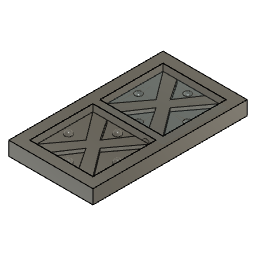
Verkefni_5_1 v3 (Autodesk Fusion 360 design; units mm, degrees)
Autodesk Fusion 360 part; units mm, degrees
sketch "Sketch1" plane through (0, 0, 0) normal (0, 0, 1) x (1, 0, 0)
  line L0 (-40, -40) -> (-10, 0)
  line L1 (-20, -40) -> (0, -10)
  line L2 (0, -10) -> (20, -40)
  line L3 (-40, -40) -> (-20, -40)
  line L4 (10, 0) -> (40, -40)
  line L5 (40, -40) -> (20, -40)
  line L6 (-40, 40) -> (-10, 0)
  line L7 (-20, 40) -> (0, 10)
  line L8 (20, 40) -> (0, 10)
  line L9 (40, 40) -> (10, 0)
  line L10 (-40, 40) -> (-20, 40)
  line L11 (20, 40) -> (40, 40)
  constraint horizontal L3
  constraint horizontal L10
  constraint parallel L10 L11
extrude "Extrude1" add sketch "Sketch1" along normal blind 5 and the other way blind 5 makes body 1
ref_plane "WorkPlane1" through (0, 0, 0) normal (0, 0, 1) x (1, 0, 0)
sketch "Sketch2" plane through (0, 0, 0) normal (0, 0, 1) x (1, 0, 0)
  line L0 (45, 45) -> (-45, 45)
  line L1 (-45, 45) -> (-45, -45)
  line L2 (-45, -45) -> (45, -45)
  line L3 (45, -45) -> (45, 45)
  line L4 (45, 45) -> (-45, -45) construction
  line L5 (-45, 45) -> (45, -45) construction
  constraint horizontal L0
  constraint perpendicular L0 L1
  constraint parallel L0 L2
  constraint parallel L1 L3
  constraint coincident L4 origin
  constraint coincident L5 origin
extrude "Extrude2" add sketch "Sketch2" along normal blind 10 and the other way blind 10 separate body makes body 2
ref_plane "WorkPlane2" through (0, 0, 0) normal (0, 0, 1) x (1, 0, 0)
split "Split1" by plane through (0, 0, 0) normal (0, 0, 1) bodies 2 makes body 3 at (-15, 15, 10)
combine "Combine1" operation cut target body 2 tool bodies 1 keep tools result as body 4 in component "Component"
combine "Combine1'" operation cut target body 3 tool bodies 1 keep tools result as body 5 in component "Component'"
sketch "Sketch3" plane through (0, 0, 0) normal (0, 0, -1) x (1, 0, 0)
  line L0 (-20, -40) -> (-40, -40)
  line L1 (-40, -40) -> (-10, 0)
  line L2 (-10, 0) -> (-40, 40)
  line L3 (-40, 40) -> (-20, 40)
  line L4 (-20, 40) -> (0, 10)
  line L5 (0, 10) -> (20, 40)
  line L6 (20, 40) -> (40, 40)
  line L7 (40, 40) -> (10, 0)
  line L8 (10, 0) -> (40, -40)
  line L9 (40, -40) -> (20, -40)
  line L10 (20, -40) -> (0, -10)
  line L11 (0, -10) -> (-20, -40)
  line L12 (45, 45) -> (-45, 45)
  line L13 (-45, 45) -> (-45, -45)
  line L14 (-45, -45) -> (45, -45)
  line L15 (45, -45) -> (45, 45)
sphere "SpherePrimitive1" add diameter 10 placed x (1, 0, 0) y (0, -1, 0) z (0, 0, -1) at (0, -35, 0) bodies 5 in component "Component'"
sphere "SpherePrimitive2" add diameter 10 placed x (1, 0, 0) y (0, -1, 0) z (0, 0, -1) at (35, 0, 0) bodies 5 in component "Component'"
sphere "SpherePrimitive3" add diameter 10 placed x (1, 0, 0) y (0, -1, 0) z (0, 0, -1) at (0, 35, 0) bodies 5 in component "Component'"
sphere "SpherePrimitive4" add diameter 10 placed x (1, 0, 0) y (0, -1, 0) z (0, 0, -1) at (-35, 0, 0) bodies 5 in component "Component'"
combine "Combine1''" operation cut target body 4 tool bodies 5 keep tools result as body 6 in component "Component''"
hole "Hole1" at (30.8553, -45, 0.457) direction (0, 1, 0) diameter 3 depth 10 tip angle 118 countersink diameter 10 countersink angle 90 bodies 5 in component "Component'"
hole "Hole1'" at (30.8553, -45, 0.457) direction (0, 1, 0) diameter 3 depth 10 tip angle 118 countersink diameter 10 countersink angle 90 bodies 6 in component "Component''"
move_body "Move1" bodies 6 to x (1, 0, 0) y (0, 1, 0) z (0, 0, 1) at (0, 10, 0) in component "Component''"
sketch "Sketch7" plane through (0, 0, 0) normal (0, 0, -1) x (1, 0, 0)
  line L0 (60, 160) -> (-60, 160)
  line L1 (-60, 160) -> (-60, -60)
  line L2 (-60, -60) -> (60, -60)
  line L3 (60, -60) -> (60, 160)
  line L4 (60, 160) -> (-60, -60) construction
  line L5 (-60, 160) -> (60, -60) construction
  point P0 (0, 50)
  constraint horizontal L0
  constraint perpendicular L0 L1
  constraint parallel L0 L2
  constraint parallel L1 L3
  constraint coincident L4 P0
  constraint coincident L5 P0
extrude "Extrude1'" add sketch "Sketch7" along normal blind 10 and the other way blind 10 separate body makes body 7 in component "Component'''"
combine "Combine1'''" operation cut target body 7 tool bodies 5 6 body 6 seen with x (1, 0, 0) y (0, -1, 0) z (0, 0, -1) at (0, -90, 0) keep tools result as body 8 in component "Component''''"
component "Component" placed x (1, 0, 0) y (0, 1, 0) z (0, 0, 1) at (0, 0, 0)
component "Component'" placed x (1, 0, 0) y (0, 1, 0) z (0, 0, 1) at (0, 0, 0)
component "Component''" placed x (1, 0, 0) y (0, -1, 0) z (0, 0, -1) at (0, -90, 0)
component "Component'''" placed x (1, 0, 0) y (0, 1, 0) z (0, 0, 1) at (0, 0, 0)
component "Component''''" placed x (1, 0, 0) y (0, 1, 0) z (0, 0, 1) at (0, 0, 0)
hidden bodies 1 2 3 4
named bodies: "X-ið"
